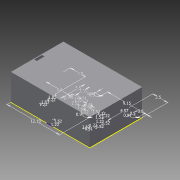
# Autodesk Inventor part: SNL_FM
Saved by Autodesk Inventor 2013 SP2 (Build 170200200, 200)
## iProperties
Created: 2006-04-26
Part Number: SNL_FM
Document SubType Name: Modeling
Designer: mcgratta
Material: Generic
Density: 1 g/cm^3
Author: mcgratta
Autodesk Inventor part; units mm, degrees
ref_plane "YZ Plane" through (0, 0, 0) normal (1, 0, 0) x (0, 1, 0)
ref_plane "XZ Plane" through (0, 0, 0) normal (0, 1, 0) x (-1, 0, 0)
ref_plane "XY Plane" through (0, 0, 0) normal (0, 0, 1) x (1, 0, 0)
sketch "Sketch1" plane through (0, 0, 0) normal (0, 0, 1) x (1, 0, 0)
  line L0 (-38.9229, 19.3084) -> (18241.0771, 19.3084)
  line L1 (18241.0771, 19.3084) -> (18241.0771, -12170.6916)
  line L2 (18241.0771, -12170.6916) -> (-38.9229, -12170.6916)
  line L3 (-38.9229, -12170.6916) -> (-38.9229, 19.3084)
  dimension "d0" = 18280
  dimension "d1" = 12190
  constraints: 8 end point, 2 parallel, 1 horizontal, 1 perpendicular
  measures "d0" distance of L0.start L0.end
  measures "d1" distance of L2.end L0.start
extrude "Extrusion1" add sketch "Sketch1" along normal blind 6100
sketch "Sketch2" plane through (0, 0, 6100) normal (0, 0, 1) x (1, 0, 0)
  line L0 (18241.0771, 19.3084) -> (18241.0771, -12170.6916) projected
  line L1 (-38.9229, 19.3084) -> (18241.0771, 19.3084) projected
  line L2 (-38.9229, -12170.6916) -> (-38.9229, 19.3084) projected
  line L3 (18241.0771, -12170.6916) -> (-38.9229, -12170.6916) projected
  line L4 (163.0061, -5175.6916) -> (763.0061, -5175.6916)
  line L5 (763.0061, -5175.6916) -> (763.0061, -6975.6916)
  line L6 (763.0061, -6975.6916) -> (163.0061, -6975.6916)
  line L7 (163.0061, -6975.6916) -> (163.0061, -5175.6916)
  line L8 (2711.0771, -2730.6916) -> (3311.0771, -2730.6916)
  line L9 (3311.0771, -2730.6916) -> (3311.0771, -3330.6916)
  line L10 (3311.0771, -3330.6916) -> (2711.0771, -3330.6916)
  line L11 (2711.0771, -3330.6916) -> (2711.0771, -2730.6916)
  line L12 (8801.0771, -2730.6916) -> (9401.0771, -2730.6916)
  line L13 (9401.0771, -2730.6916) -> (9401.0771, -3330.6916)
  line L14 (9401.0771, -3330.6916) -> (8801.0771, -3330.6916)
  line L15 (8801.0771, -3330.6916) -> (8801.0771, -2730.6916)
  line L16 (14891.0771, -2730.6916) -> (15491.0771, -2730.6916)
  line L17 (15491.0771, -2730.6916) -> (15491.0771, -3330.6916)
  line L18 (15491.0771, -3330.6916) -> (14891.0771, -3330.6916)
  line L19 (14891.0771, -3330.6916) -> (14891.0771, -2730.6916)
  line L20 (2711.0771, -8820.6916) -> (3311.0771, -8820.6916)
  line L21 (3311.0771, -8820.6916) -> (3311.0771, -9420.6916)
  line L22 (3311.0771, -9420.6916) -> (2711.0771, -9420.6916)
  line L23 (2711.0771, -9420.6916) -> (2711.0771, -8820.6916)
  line L24 (8801.0771, -8820.6916) -> (9401.0771, -8820.6916)
  line L25 (9401.0771, -8820.6916) -> (9401.0771, -9420.6916)
  line L26 (9401.0771, -9420.6916) -> (8801.0771, -9420.6916)
  line L27 (8801.0771, -9420.6916) -> (8801.0771, -8820.6916)
  line L28 (14891.0771, -8820.6916) -> (15491.0771, -8820.6916)
  line L29 (15491.0771, -8820.6916) -> (15491.0771, -9420.6916)
  line L30 (15491.0771, -9420.6916) -> (14891.0771, -9420.6916)
  line L31 (14891.0771, -9420.6916) -> (14891.0771, -8820.6916)
  dimension "d4" = 600
  dimension "d5" = 600
  dimension "d6" = 2750
  dimension "d7" = 600
  dimension "d8" = 600
  dimension "d9" = 2750
  dimension "d10" = 2750
  dimension "d11" = 600
  dimension "d12" = 600
  dimension "d13" = 2750
  dimension "d14" = 2750
  dimension "d15" = 8840
  dimension "d16" = 600
  dimension "d17" = 600
  dimension "d18" = 2750
  dimension "d19" = 2750
  dimension "d20" = 600
  dimension "d21" = 600
  dimension "d22" = 2750
  dimension "d23" = 600
  dimension "d24" = 600
  dimension "d25" = 2750
  dimension "d26" = 2750
  dimension "d27" = 8840
  dimension "d28" = 1800
  dimension "d29" = 600
  dimension "d30" = 5195
  constraints: 56 end point, 14 parallel, 7 horizontal, 7 perpendicular
  measures "d4" distance of L8.end L9.end
  measures "d5" distance of L8.start L8.end
  measures "d6" distance between parallel lines of L2 L11
  measures "d7" distance of L12.start L12.end
  measures "d8" distance of L12.end L13.end
  measures "d9" distance between parallel lines of L1 L8
  measures "d10" distance between parallel lines of L1 L12
  measures "d11" distance of L18.end L16.start
  measures "d12" distance of L16.start L16.end
  measures "d13" distance between parallel lines of L1 L16
  measures "d14" distance between parallel lines of L0 L17
  measures "d15" distance between parallel lines of L0 L13
  measures "d16" distance of L22.end L20.start
  measures "d17" distance of L20.start L20.end
  measures "d18" distance between parallel lines of L3 L22
  measures "d19" distance between parallel lines of L2 L23
  measures "d20" distance of L26.end L24.start
  measures "d21" distance of L24.start L24.end
  measures "d22" distance between parallel lines of L3 L26
  measures "d23" distance of L30.end L28.start
  measures "d24" distance of L28.start L28.end
  measures "d25" distance between parallel lines of L3 L30
  measures "d26" distance between parallel lines of L0 L29
  measures "d27" distance between parallel lines of L0 L25
  measures "d28" distance of L4.end L5.end
  measures "d29" distance of L4.start L4.end
  measures "d30" distance between parallel lines of L3 L6
shell "Shell1" thickness 1 removed faces 0
extrude "Extrusion2" cut sketch "Sketch2" against normal mid plane 1000 contours L4 L5 L6 L7
extrude "Extrusion3" add sketch "Sketch2" against normal blind 1200 contours L20 L21 L22 L23
extrude "Extrusion4" add sketch "Sketch2" against normal blind 1200 contours L24 L25 L26 L27
extrude "Extrusion5" add sketch "Sketch2" against normal blind 1200 contours L28 L29 L30 L31
extrude "Extrusion6" add sketch "Sketch2" against normal blind 1200 contours L8 L9 L10 L11
extrude "Extrusion7" add sketch "Sketch2" against normal blind 1200 contours L12 L13 L14 L15
extrude "Extrusion8" add sketch "Sketch2" against normal blind 1200 contours L16 L17 L18 L19
sketch "Sketch5" plane through (0, 0, 0) normal (0, 0, -1) x (-1, 0, 0)
  line L0 (38.9229, 19.3084) -> (-18241.0771, 19.3084) projected
  line L1 (-18241.0771, 19.3084) -> (-18241.0771, -12170.6916) projected
  line L2 (-18241.0771, -12170.6916) -> (38.9229, -12170.6916) projected
  line L3 (38.9229, -12170.6916) -> (38.9229, 19.3084) projected
  line L4 (-6981.0771, -3330.6916) -> (-5761.0771, -3330.6916)
  line L5 (-5761.0771, -3330.6916) -> (-5761.0771, -5310.6916)
  line L6 (-5761.0771, -5310.6916) -> (-6981.0771, -5310.6916)
  line L7 (-6981.0771, -5310.6916) -> (-6981.0771, -3330.6916)
  line L8 (-6981.0771, -3330.6916) -> (-8501.0771, -3330.6916)
  line L9 (-8501.0771, -3330.6916) -> (-8501.0771, -4550.6916)
  line L10 (-8501.0771, -4550.6916) -> (-6981.0771, -4550.6916)
  line L11 (-6981.0771, -4550.6916) -> (-6981.0771, -3330.6916)
  line L12 (-8501.0771, -3330.6916) -> (-9721.0771, -3330.6916)
  line L13 (-9721.0771, -3330.6916) -> (-9721.0771, -5310.6916)
  line L14 (-9721.0771, -5310.6916) -> (-8501.0771, -5310.6916)
  line L15 (-8501.0771, -5310.6916) -> (-8501.0771, -3330.6916)
  line L16 (-9721.0771, -3330.6916) -> (-10941.0771, -3330.6916)
  line L17 (-10941.0771, -3330.6916) -> (-10941.0771, -5300)
  line L18 (-10941.0771, -5300) -> (-9721.0771, -5300)
  line L19 (-9721.0771, -5300) -> (-9721.0771, -3330.6916)
  line L20 (-10941.0771, -3330.6916) -> (-12461.0771, -3330.6916)
  line L21 (-12461.0771, -3330.6916) -> (-12461.0771, -4550.6916)
  line L22 (-12461.0771, -4550.6916) -> (-10941.0771, -4550.6916)
  line L23 (-10941.0771, -4550.6916) -> (-10941.0771, -3330.6916)
  line L24 (-12461.0771, -3330.6916) -> (-13981.0771, -3330.6916)
  line L25 (-13981.0771, -3330.6916) -> (-13981.0771, -4550.6916)
  line L26 (-13981.0771, -4550.6916) -> (-12461.0771, -4550.6916)
  line L27 (-12461.0771, -4550.6916) -> (-12461.0771, -3330.6916)
  line L28 (-14741.0771, -4550.6916) -> (-13521.0771, -4550.6916)
  line L29 (-13521.0771, -4550.6916) -> (-13521.0771, -6070.6916)
  line L30 (-13521.0771, -6070.6916) -> (-14741.0771, -6070.6916)
  line L31 (-14741.0771, -6070.6916) -> (-14741.0771, -4550.6916)
  line L32 (-14741.0771, -6070.6916) -> (-13521.0771, -6070.6916)
  line L33 (-13521.0771, -6070.6916) -> (-13521.0771, -7590.6916)
  line L34 (-13521.0771, -7590.6916) -> (-14741.0771, -7590.6916)
  line L35 (-14741.0771, -7590.6916) -> (-14741.0771, -6070.6916)
  line L36 (-14741.0771, -7590.6916) -> (-13831.0771, -7590.6916)
  line L37 (-13831.0771, -7590.6916) -> (-13831.0771, -9110.6916)
  line L38 (-13831.0771, -9110.6916) -> (-14741.0771, -9110.6916)
  line L39 (-14741.0771, -9110.6916) -> (-14741.0771, -7590.6916)
  line L40 (-9800, -10950.6916) -> (-8280, -10950.6916)
  line L41 (-8280, -10950.6916) -> (-8280, -12170.6916)
  line L42 (-8280, -12170.6916) -> (-9800, -12170.6916)
  line L43 (-9800, -12170.6916) -> (-9800, -10950.6916)
  line L44 (-3461.0771, -5480.6916) -> (-4681.0771, -5480.6916)
  line L45 (-4681.0771, -5480.6916) -> (-4681.0771, -7310.6916)
  line L46 (-4681.0771, -7310.6916) -> (-3461.0771, -7310.6916)
  line L47 (-3461.0771, -7310.6916) -> (-3461.0771, -5480.6916)
  line L48 (-3461.0771, -7310.6916) -> (-4681.0771, -7310.6916)
  line L49 (-4681.0771, -7310.6916) -> (-4681.0771, -9140.6916)
  line L50 (-4681.0771, -9140.6916) -> (-3461.0771, -9140.6916)
  line L51 (-3461.0771, -9140.6916) -> (-3461.0771, -7310.6916)
  line L52 (-4681.0771, -5480.6916) -> (-5761.0771, -4320.6916)
  line L53 (-4681.0771, -5480.6916) -> (-3627.7417, -4500)
  line L54 (-3627.7417, -4500) -> (-4700.1477, -3348.1566)
  line L55 (-4700.1477, -3348.1566) -> (-5761.0771, -4320.6916)
  circle A0 centre (-12151.0771, -6070.6916) radius 455
  circle A1 centre (-9111.0771, -4300) radius 455
  circle A2 centre (-9091.0771, -480.6916) radius 455
  circle A3 centre (-17741.0771, -480.6916) radius 455
  dimension "d66" = 1220
  dimension "d67" = 1980
  dimension "d68" = 3350
  dimension "d69" = 5800
  dimension "d70" = 1520
  dimension "d71" = 1220
  dimension "d72" = 1220
  dimension "d73" = 1980
  dimension "d74" = 1220
  dimension "d75" = 1520
  dimension "d76" = 1220
  dimension "d77" = 1520
  dimension "d78" = 1520
  dimension "d79" = 1220
  dimension "d80" = 3500
  dimension "d81" = 4570
  dimension "d82" = 1220
  dimension "d83" = 1520
  dimension "d84" = 1220
  dimension "d85" = 1520
  dimension "d86" = 910
  dimension "d90" = 1520
  dimension "d91" = 1220
  dimension "d92" = 1830
  dimension "d93" = 1220
  dimension "d94" = 3500
  dimension "d95" = 5500
  dimension "d96" = 1830
  dimension "d97" = 1220
  dimension "d126" = 910
  dimension "d128" = 12190
  dimension "d129" = 910
  dimension "d130" = 610
  dimension "d137" = 910
  dimension "d138" = 9150
  dimension "d139" = 910
  dimension "d140" = 500
  dimension "d141" = 500
  dimension "d142" = 500
  constraints: 104 end point, 24 parallel, 14 perpendicular, 12 horizontal, 4 centre point, 1 midpoint, 1 point on line
  measures "d66" distance of L4.start L4.end
  measures "d67" distance of L4.end L5.end
  measures "d68" distance between parallel lines of L0 L4
  measures "d69" distance between parallel lines of L3 L5
  measures "d70" distance of L9.end L10.end
  measures "d71" distance of L10.end L4.start
  measures "d72" distance of L13.end L14.end
  measures "d73" distance of L12.end L13.end
  measures "d74" distance of L17.end L18.end
  measures "d75" distance of L21.end L22.end
  measures "d76" distance of L20.end L21.end
  measures "d77" distance of L25.end L26.end
  measures "d78" distance of L30.end L28.start
  measures "d79" distance of L29.end L30.end
  measures "d80" distance between parallel lines of L1 L31
  measures "d81" distance between parallel lines of L0 L28
  measures "d82" distance of L24.end L25.end
  measures "d83" distance of L34.end L30.end
  measures "d84" distance of L33.end L34.end
  measures "d85" distance of L36.end L37.end
  measures "d86" distance of L37.end L38.end
  measures "d90" distance of L40.start L40.end
  measures "d91" distance of L42.end L40.start
  measures "d92" distance of L46.end L44.start
  measures "d93" distance of L45.end L46.end
  measures "d94" distance between parallel lines of L3 L47
  measures "d95" distance between parallel lines of L0 L44
  measures "d96" distance of L50.end L46.end
  measures "d97" distance of L49.end L50.end
  measures "d126" diameter of A0
  measures "d128" distance from line of L3 A0.centre
  measures "d129" diameter of A1
  measures "d130" distance from line of L19 A1.centre
  measures "d137" diameter of A2
  measures "d138" distance from line of L1 A2.centre
  measures "d139" diameter of A3
  measures "d140" distance from line of L0 A3.centre
  measures "d141" distance from line of L1 A3.centre
  measures "d142" distance from line of L0 A2.centre
extrude "Extrusion23" add sketch "Sketch5" against normal blind 10 contours A0
extrude "Extrusion26" add sketch "Sketch5" against normal blind 10 contours A2
extrude "Extrusion27" add sketch "Sketch5" against normal blind 10 contours A3
body "Solid1"
